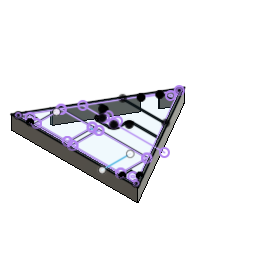
krabicka (Autodesk Fusion 360 design; units mm, degrees)
Autodesk Fusion 360 part; units mm, degrees
sketch "Sketch1" plane through (0, 0, 0) normal (0, 1, 0) x (1, 0, 0) in component "deska"
  line L0 (0, 0) -> (95, 0)
  line L1 (95, 0) -> (47.5, 82.2724)
  line L2 (47.5, 82.2724) -> (0, 0)
  line L3 (23.75, 41.1362) -> (95, 0) construction
  line L4 (0, 0) -> (71.25, 41.1362) construction
  circle A0 centre (95, 0) radius 7.02 construction
  circle A1 centre (47.5, 82.2724) radius 7.02 construction
  circle A2 centre (0, 0) radius 7.02 construction
  line L5 (47.5, 82.2724) -> (47.5, 0) construction
  circle A3 centre (47.5, 75.2524) radius 1
  circle A4 centre (6.0795, 3.51) radius 1
  circle A5 centre (88.9205, 3.51) radius 1
  line L6 (81.6, 8.0217) -> (81.6, -11.5309) construction
  line L7 (81.6, 1) -> (43, 1)
  line L8 (43, 1) -> (43, 22)
  line L9 (43, 22) -> (81.6, 22)
  line L10 (81.6, 22) -> (81.6, 1)
  line L11 (38, 22) -> (38, -18.5027) construction
  line L12 (38, 1.6) -> (13, 1.6)
  line L13 (13, 1.6) -> (13, 21.6)
  line L14 (13, 21.6) -> (38, 21.6)
  line L15 (38, 21.6) -> (38, 1.6)
  line L16 (19.0526, 33) -> (84.8076, 33) construction
  line L17 (36.5526, 33) -> (44.0526, 33)
  line L18 (44.0526, 33) -> (44.0526, 36)
  line L19 (44.0526, 36) -> (36.5526, 36)
  line L20 (36.5526, 36) -> (36.5526, 33)
  line L21 (47.5, 44.7724) -> (25.8494, 44.7724) construction
  line L22 (44.25, 44.7724) -> (50.75, 44.7724)
  line L23 (50.75, 44.7724) -> (50.75, 50.7724)
  line L24 (50.75, 50.7724) -> (44.25, 50.7724)
  line L25 (44.25, 50.7724) -> (44.25, 44.7724)
  line L26 (38.55, 44.7724) -> (38.55, 50.7724)
  line L27 (32.05, 50.7724) -> (32.05, 44.7724)
  line L28 (38.55, 50.7724) -> (32.05, 50.7724)
  line L29 (32.05, 44.7724) -> (38.55, 44.7724)
  line L30 (62.95, 44.7724) -> (62.95, 50.7724)
  line L31 (56.45, 50.7724) -> (56.45, 44.7724)
  line L32 (62.95, 50.7724) -> (56.45, 50.7724)
  line L33 (56.45, 44.7724) -> (62.95, 44.7724)
  line L34 (47.5, 82.2724) -> (31, 82.2724) construction
  line L35 (47.5, 82.2724) -> (63, 82.2724) construction
  line L36 (49.5, 54.6724) -> (55.1, 64.3724)
  line L37 (55.1, 64.3724) -> (42.4, 71.6724)
  line L38 (42.4, 71.6724) -> (36.9, 62.0724)
  line L39 (36.9, 62.0724) -> (49.5, 54.6724)
  point P0 (36.9, 62.0724)
  point P1 (42.4, 71.6724)
  point P2 (55.1, 64.3724)
  point P3 (49.5, 54.6724)
  dimension "d1" = 95
  dimension "d2" = 95
  dimension "d3" = 95
  dimension "d4" = 14.04
  dimension "d5" = 2
  dimension "d6" = 2
  dimension "d7" = 2
  dimension "d13" = 13.4
  dimension "d14" = 38.6
  dimension "d16" = 21
  dimension "d17" = 38
  dimension "d18" = 1
  dimension "d19" = 25
  dimension "d20" = 20
  dimension "d21" = 1.6
  dimension "d22" = 33
  dimension "d23" = 3
  dimension "d24" = 7.5
  dimension "d25" = 17.5
  dimension "d26" = 37.5
  dimension "d27" = 6.5
  dimension "d28" = 6
  dimension "d29" = 3.25
  dimension "d32" = 12.2
  dimension "d33" = 0
  dimension "d34" = 10.6
  dimension "d35" = 5.1
  dimension "d36" = 20.2
  dimension "d37" = 10.6
  dimension "d38" = 7.6
  dimension "d39" = 17.9
  dimension "d40" = 27.6
  dimension "d41" = 2
  constraint coincident L0.start L2.end
  constraint horizontal L0
  constraint midpoint L2 L3.start
  constraint midpoint L1 L4.end
  constraint coincident L0.end L1.start
  constraint coincident L1.end L2.start
  constraint equal A0 A2
  constraint equal A0 A1
  constraint midpoint L0 L5.end
  constraint coincident A1 A3.centre
  constraint coincident L5 A3.centre
  constraint coincident A2 A4.centre
  constraint coincident L4 A4.centre
  constraint coincident A0 A5.centre
  constraint coincident L3 A5.centre
  constraint perpendicular L0 L6
  constraint horizontal L7
  constraint vertical L8
  constraint horizontal L9
  constraint vertical L10
  constraint coincident L6 L7.start
  constraint vertical L11
  constraint horizontal L12
  constraint vertical L13
  constraint horizontal L14
  constraint vertical L15
  constraint coincident L11 L12.start
  constraint horizontal L16
  constraint horizontal L17
  constraint vertical L18
  constraint horizontal L19
  constraint vertical L20
  constraint coincident L16 L17.start
  constraint coincident L2 L16.start
  constraint coincident L5 L21.start
  constraint perpendicular L5 L21
  constraint coincident L2 L21.end
  constraint horizontal L22
  constraint vertical L23
  constraint horizontal L24
  constraint vertical L25
  constraint coincident L21 L22.start
  constraint perpendicular L5 L34
  constraint parallel L34 L35
  constraint coincident P3 L36.start
  constraint coincident P2 L36.end
  constraint coincident P1 L37.end
  constraint coincident P0 L38.end
  measures "d1" distance of L0.start L0.end
  measures "d2" distance of L0.end L1.end
  measures "d3" distance of L1.end L0.start
  measures "d4" diameter of A0
  measures "d5" diameter of A3
  measures "d6" diameter of A4
  measures "d7" diameter of A5
  measures "d13" distance of L0.end L6
  measures "d14" distance of L8.end L9.end
  measures "d16" distance of L7.end L8.end
  measures "d17" distance of L0.start L11
  measures "d18" distance of L0 L7
  measures "d19" distance of L13.end L14.end
  measures "d20" distance of L12.end L13.end
  measures "d21" distance of L0 L12
  measures "d22" distance of L0 L16
  measures "d23" distance of L17.start L19.end
  measures "d24" distance of L18.end L19.end
  measures "d25" distance of L16.start L17.start
  measures "d26" distance of L1.end L21
  measures "d27" distance of L23.end L24.end
  measures "d28" distance of L22.start L24.end
  measures "d29" distance of L5 L25
  measures "d34" distance of P1 L34
  measures "d35" distance of L5 P1
  measures "d36" distance of P0 L34
  measures "d37" distance of L5 P0
  measures "d38" distance of L5 P2
  measures "d39" distance of P2 L35
  measures "d40" distance of P3 L35
  measures "d41" distance of L5 P3
extrude "Extrude1" add sketch "Sketch1" along normal blind 1.6 contours L0 L1 L2 | L7 L8 L9 L10 | L12 L13 L14 L15 | L17 L18 L19 L20 | L22 L23 L24 L25 | L26 L27 L28 L29 | L30 L31 L32 L33 | L36 L37 L38 L39 makes body 1 in component "deska"
ref_plane "WorkPlane1" through (47.5, 11.1, -41.1362) normal (0, 1, 0) x (1, 0, 0) in component "krabicka"
sketch "Sketch1 (2)" plane through (47.5, 11.1, -41.1362) normal (0, 1, 0) x (1, 0, 0) in component "krabicka"
  circle A0 centre (-41.4205, -37.6262) radius 1
  circle A1 centre (0, 34.1162) radius 1
  circle A2 centre (41.4205, -37.6262) radius 1
  line L0 (0, 41.1362) -> (-47.5, -41.1362)
  line L1 (-47.5, -41.1362) -> (47.5, -41.1362)
  line L2 (47.5, -41.1362) -> (0, 41.1362)
  line L3 (48.366, -41.6362) -> (0, 42.1362)
  line L4 (0, 42.1362) -> (-48.366, -41.6362)
  line L5 (-48.366, -41.6362) -> (48.366, -41.6362)
  line L6 (-50.9641, -43.1362) -> (50.9641, -43.1362)
  line L7 (50.9641, -43.1362) -> (0, 45.1362)
  line L8 (0, 45.1362) -> (-50.9641, -43.1362)
  line L9 (24.4899, -22.8742) -> (24.4899, -45.5)
  line L10 (-44.9597, -35.7362) -> (-37.9597, -35.7362)
  line L11 (-37.9597, -35.7362) -> (-37.9597, -41.1362)
  line L12 (36.4585, -41.1362) -> (36.4585, -34.1362)
  line L13 (36.4585, -34.1362) -> (43.4585, -34.1362)
  line L14 (-5.7735, 32.1362) -> (5.7735, 32.1362)
  line L15 (-17.3205, 12.1362) -> (17.3205, 12.1362)
  line L16 (-24.183, 0.25) -> (-17.9474, 0.25)
  line L17 (-14.9474, -2.75) -> (-14.9474, -9.1362)
  line L18 (-11.9474, -12.1362) -> (-2.4474, -12.1362)
  line L19 (0.5526, -9.1362) -> (0.5526, -2.75)
  line L20 (3.5526, 0.25) -> (24.183, 0.25)
  arc A3 (-14.9474, -2.75) -> (-17.9474, 0.25) centre (-17.9474, -2.75) ccw
  arc A4 (3.5526, 0.25) -> (0.5526, -2.75) centre (3.5526, -2.75) ccw
  arc A5 (-14.9474, -9.1362) -> (-11.9474, -12.1362) centre (-11.9474, -9.1362) ccw
  arc A6 (-2.4474, -12.1362) -> (0.5526, -9.1362) centre (-2.4474, -9.1362) ccw
  line L21 (-10.9474, -5.1362) -> (-10.9474, -8.1362)
  line L22 (-3.4474, -8.1362) -> (-3.4474, -5.1362)
  line L23 (-28.4474, -8.1362) -> (37.3076, -8.1362)
  line L24 (-5.1, 30.5362) -> (-10.6, 20.9362)
  line L25 (-10.6, 20.9362) -> (-13.1289, 22.3963)
  line L26 (-5.1, 30.5362) -> (-7.597, 31.9778)
  line L27 (-34.5, -19.5362) -> (-9.5, -19.5362)
  line L28 (-39.5326, -23.3362) -> (-34.4423, -23.3362)
  line L29 (-44.9597, -35.7362) -> (-46.6917, -35.7362)
  line L30 (-9.5, -19.5362) -> (-9.5, -39.5362)
  line L31 (-9.5, -39.5362) -> (-34.5, -39.5362)
  line L32 (-34.5, -39.5362) -> (-34.5, -19.5362)
  line L33 (-35, -40.0362) -> (-35, -19.0362)
  line L34 (-35, -19.0362) -> (-9, -19.0362)
  line L35 (-9, -19.0362) -> (-9, -40.0362)
  line L36 (-9, -40.0362) -> (-35, -40.0362)
  line L37 (-4.5, -19.1362) -> (34.1, -19.1362)
  line L38 (-4.5, -40.1362) -> (-4.5, -19.1362)
  line L39 (34.1, -19.1362) -> (34.1, -40.1362)
  line L40 (34.1, -40.1362) -> (-4.5, -40.1362)
  line L41 (-5, -40.6362) -> (-5, -18.6362)
  line L42 (-5, -18.6362) -> (34.6, -18.6362)
  line L43 (34.6, -18.6362) -> (34.6, -40.6362)
  line L44 (34.6, -40.6362) -> (-5, -40.6362)
  line L45 (-9, -20.9386) -> (-5, -20.9386)
  line L46 (-24.183, -0.75) -> (-17.9474, -0.75)
  arc A7 (-15.9474, -2.75) -> (-17.9474, -0.75) centre (-17.9474, -2.75) ccw
  line L47 (-15.9474, -2.75) -> (-15.9474, -9.1362)
  arc A8 (-15.9474, -9.1362) -> (-11.9474, -13.1362) centre (-11.9474, -9.1362) ccw
  line L48 (-11.9474, -13.1362) -> (-2.4474, -13.1362)
  arc A9 (-2.4474, -13.1362) -> (1.5526, -9.1362) centre (-2.4474, -9.1362) ccw
  line L49 (1.5526, -9.1362) -> (1.5526, -2.75)
  arc A10 (3.5526, -0.75) -> (1.5526, -2.75) centre (3.5526, -2.75) ccw
  line L50 (3.5526, -0.75) -> (24.183, -0.75)
  line L51 (-17.3205, 12.8862) -> (17.3205, 12.8862)
  line L52 (-24.183, -0.75) -> (-24.7604, -0.75)
  line L53 (24.183, -0.75) -> (24.7604, -0.75)
  line L54 (-37.9597, -41.1362) -> (-37.9597, -41.6362)
  line L55 (36.4585, -41.1362) -> (36.4585, -41.6362)
  line L56 (44.0359, -34.1362) -> (43.4585, -34.1362)
  point P0 (0, 41.1362)
  dimension "d11" = 0.5
  dimension "d12" = 2
  dimension "d58" = 5.4
  dimension "d59" = 7
  dimension "d60" = 7
  dimension "d61" = 7
  dimension "d62" = 9
  dimension "d63" = 30
  dimension "d64" = 3
  dimension "d65" = 4
  dimension "d66" = 4
  dimension "d67" = 4
  dimension "d68" = 3.8
  dimension "d73" = -0.5
  dimension "d74" = -0.5
  dimension "d75" = 1
  dimension "d76" = -0.75
  constraint vertical L9
  constraint coincident L4 L10.start
  constraint horizontal L10
  constraint coincident L1 L11.end
  constraint perpendicular L1 L11
  constraint coincident L1 L12.start
  constraint perpendicular L1 L12
  constraint coincident L2 L13.end
  constraint perpendicular L12 L13
  constraint coincident L4 L14.start
  constraint coincident L3 L14.end
  constraint horizontal L14
  constraint coincident L4 L15.start
  constraint coincident L3 L15.end
  constraint horizontal L15
  constraint midpoint L4 L16.start
  constraint horizontal L16
  constraint perpendicular L16 L17
  constraint perpendicular L17 L18
  constraint perpendicular L18 L19
  constraint coincident L3 L20.end
  constraint perpendicular L19 L20
  constraint tangent L16 A3
  constraint tangent L17 A3
  constraint tangent L19 A4
  constraint tangent L20 A4
  constraint equal A3 A4
  constraint tangent L17 A5
  constraint tangent L18 A5
  constraint equal A3 A5
  constraint tangent L18 A6
  constraint tangent L19 A6
  constraint equal A3 A6
  constraint collinear L16 L20
  constraint coincident L24.end L25.start
  constraint coincident L8 L25.end
  constraint perpendicular L8 L25
  constraint coincident L24.start L26.start
  constraint coincident L8 L26.end
  constraint perpendicular L8 L26
  constraint coincident L8 L28.start
  constraint horizontal L28
  constraint coincident L8 L29.end
  constraint parallel L10 L29
  constraint coincident L35 L45.start
  constraint coincident L41 L45.end
  constraint perpendicular L41 L45
  constraint coincident L4 L52.end
  constraint parallel L46 L52
  constraint coincident L3 L53.end
  constraint perpendicular L49 L53
  constraint coincident L5 L54.end
  constraint perpendicular L5 L54
  constraint coincident L5 L55.end
  constraint perpendicular L5 L55
  constraint coincident L3 L56.start
  measures "d58" distance of L10.end L11.end
  measures "d59" distance of L10.start L10.end
  measures "d60" distance of L12.end L13.end
  measures "d61" distance of L12.start L12.end
  measures "d62" distance of L14 P0
  measures "d63" distance of L3.end L15
  measures "d64" radius of A3
  measures "d65" distance of L17 L21
  measures "d66" distance of L19 L22
  measures "d67" distance of L18 L23
  measures "d68" distance of L27 L28
extrude "Extrude2" add sketch "Sketch1" along normal blind 4.2 contours L36 L37 L38 L39 bodies 1 in component "deska"
extrude "Extrude3" add sketch "Sketch1" along normal blind 6.45 contours L7 L8 L9 L10 bodies 1 in component "deska"
extrude "Extrude4" add sketch "Sketch1" along normal blind 6.45 contours L22 L23 L24 L25 | L26 L27 L28 L29 | L30 L31 L32 L33 bodies 1 in component "deska"
extrude "Extrude5" add sketch "Sketch1" along normal blind 5.7 contours L12 L13 L14 L15 bodies 1 in component "deska"
extrude "Extrude6" add sketch "Sketch1" along normal blind 6.45 contours L17 L18 L19 L20 bodies 1 in component "deska"
sketch "Sketch2" plane through (0, 5.7, 0) normal (0, 1, 0) x (-1, 0, 0) in component "deska"
  line L0 (-38, -21.6) -> (-13, -21.6)
  line L1 (-13, -21.6) -> (-13, -1.6)
  line L2 (-13, -1.6) -> (-38, -1.6)
  line L3 (-38, -1.6) -> (-38, -21.6)
  line L4 (-11, -15.35) -> (-21, -15.35)
  line L5 (-21, -15.35) -> (-21, -7.85)
  line L6 (-21, -7.85) -> (-11, -7.85)
  line L7 (-11, -7.85) -> (-11, -15.35)
  line L8 (-13, -1.6) -> (-13, -21.6)
  line L9 (-13, -21.6) -> (-38, -21.6)
  dimension "d52" = 10
  dimension "d53" = 7.5
  dimension "d54" = 2
  dimension "d55" = 6.25
  constraint horizontal L4
  constraint vertical L5
  constraint horizontal L6
  constraint vertical L7
  measures "d52" distance of L4.start L4.end
  measures "d53" distance of L4.start L6.end
  measures "d54" distance of L7 L8
  measures "d55" distance of L4 L9
extrude "Extrude7" add sketch "Sketch2" along normal blind 3.5 contours L1 L4 L5 L6 L8 | L1 L4 L6 L7 L8 bodies 1 in component "deska"
extrude "Extrude1'" add sketch "Sketch1 (2)" against normal blind 11 separate body contours L4 L8 L25 L28 | L4 L5 L6 L8 L9 L29 | L3 L4 L7 L8 L23 L26 | L3 L5 L6 L7 L9 L23 makes body 2 at (25.5699, 3.7667, -48.2883) makes body 3 at (30.512, 7.4333, 2) in component "krabicka"
extrude "Extrude8" add sketch "Sketch1 (2)" against normal blind 9.4 separate body contours L0 L4 L16 L52 | L0 L16 L17 A3 L23 L46 A7 L47 | L17 L18 L19 A5 A6 L23 L47 A8 L48 A9 L49 | L0 L4 L15 L51 | L0 L2 L15 L51 | L2 L3 L15 L51 | L0 L1 L4 L5 L10 L54 | L2 L3 L20 L53 | L2 L19 L20 A4 L23 L49 A10 L50 | L0 L1 L10 L11 | L0 L2 L14 | L0 L2 L3 L4 L14 | L1 L2 L3 L5 L55 L56 | L1 L2 L12 L13 makes body 4 at (45.5755, 7.9667, -73.2724) makes body 5 at (87.9277, 7.9667, 0.5) makes body 6 at (58.1218, 7.9667, -40.3862) makes body 7 at (2.6028, 7.9667, 0.5) makes body 8 at (41.7265, 7.9667, -53.2724) in component "deska"
extrude "Extrude9" add sketch "Sketch1 (2)" against normal blind 11 separate body contours L4 L8 L25 L26 makes body 9 in component "deska"
extrude "Extrude10" add sketch "Sketch1 (2)" along normal blind 1 contours L0 L23 L46 A7 L47 | L0 L4 L16 L52 | L0 L16 L17 A3 L23 L46 A7 L47 | L0 L4 L28 L33 L34 L52 | L0 L2 L23 L34 L35 L41 L42 L45 L47 A8 L48 A9 L49 | L4 L8 L25 L28 | L0 L33 L34 L35 L36 | L17 L18 L19 A5 A6 L23 L47 A8 L48 A9 L49 | L0 L4 L15 L51 | L0 L2 L15 L51 | L0 L4 L10 L28 | L4 L8 L28 L29 | L0 L28 L33 | L0 L4 L25 L51 | L0 L2 L14 L24 L25 L26 L51 | L2 L3 L15 L51 | L0 L1 L4 L5 L10 L54 | L4 L5 L6 L8 L9 L29 | L0 L1 L9 L10 L11 L28 L33 L35 L36 L41 L44 L45 | L0 L4 L25 L26 | L0 L24 L25 L26 | L2 L3 L14 L51 | L2 L3 L20 L53 | L2 L19 L20 A4 L23 L49 A10 L50 | L3 L4 L7 L8 L23 L26 | L0 L1 L10 L11 | L4 L8 L25 L26 | L2 L41 L42 L43 L44 | L0 L4 L14 L26 | L0 L2 L14 | L0 L2 L3 L4 L14 | L2 L3 L23 L53 | L2 L23 L49 A10 L50 | L1 L5 L9 L54 | L2 L3 L23 L42 L43 L56 | L1 L5 L9 L55 | L3 L5 L6 L7 L9 L23 | L1 L2 L9 L12 L13 L43 L44 | L1 L2 L3 L5 L55 L56 | L1 L2 L12 L13 | L27 L30 L31 L32 | L37 L38 L39 L40 bodies 4 5 6 7 8 9 in component "deska"
sketch "Sketch3" plane through (-1.7321, 0, -1) normal (-0.866025, 0, -0.5) x (-0.5, 0, 0.866025) in component "deska"
  line L0 (-83.2701, 11.1) -> (-83.2701, 0.1)
  line L1 (-83.2701, 0.1) -> (-72.2063, 0.1)
  line L2 (-72.2063, 0.1) -> (-72.2063, 11.1)
  line L3 (-72.2063, 11.1) -> (3.4641, 11.1)
  line L4 (3.4641, 11.1) -> (3.4641, 12.1)
  line L5 (3.4641, 12.1) -> (-98.4641, 12.1)
  line L6 (-98.4641, 12.1) -> (-98.4641, 11.1)
  line L7 (-98.4641, 11.1) -> (-83.2701, 11.1)
  line L8 (-83.2701, 6.7) -> (-72.2063, 6.7)
  line L9 (-83.2701, 1.7) -> (-72.2063, 1.7)
  dimension "d86" = 1.6
  dimension "d87" = 5
  constraint coincident L0 L8.start
  constraint coincident L2 L8.end
  constraint perpendicular L2 L8
  constraint coincident L0 L9.start
  constraint coincident L2 L9.end
  constraint horizontal L9
  measures "d86" distance of L1 L9
  measures "d87" distance of L8 L9
extrude "Extrude11" cut sketch "Sketch3" against normal up to surface (1.5 mm away) contours L0 L2 L8 L9 bodies 4 makes body 10 at (36.2151, 1.1667, -66.7263) in component "deska"
sketch "Sketch2 (2)" plane through (0, 0, -17.8) normal (0, 0, 1) x (1, 0, 0) in component "krabicka"
  line L0 (9.6995, 11.1) -> (7.9674, 11.1)
  line L1 (7.9674, 11.1) -> (7.9674, 0.1)
  line L2 (7.9674, 0.1) -> (9.6995, 0.1)
  line L3 (9.6995, 0.1) -> (9.6995, 11.1)
component "deska" placed x (1, 0, 0) y (0, 1, 0) z (0, 0, 1) at (0, 0, 0)
component "krabicka" placed x (1, 0, 0) y (0, 1, 0) z (0, 0, 1) at (0, 0, 0)
equation "d4 = ( 7.02 * 2 ) * 1 mm"
equation "d29 = ( 6.5 * 0.5 ) * 1 mm"
equation "d40 = 17.9 mm + 9.7 mm"
equation "d55 = 10 mm - 3.75 mm"
equation "d79 = -( 11 mm - 1.6 mm )"
